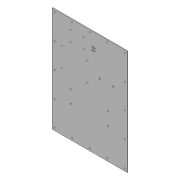
# Autodesk Inventor part: Board_Mounter
Saved by Autodesk Inventor 2020 (Build 240168000, 168)
## iProperties
Created: 2020-11-10
Part Number: Board_Mounter
Material: Generic
Document SubType Name: Modeling
Designer: magnarecta
Density: 1 g/cm^3
Appearance: Default
Author: magnarecta
Autodesk Inventor part; units mm, degrees
ref_plane "YZ Plane" through (0, 0, 0) normal (1, 0, 0) x (0, 1, 0)
ref_plane "XZ Plane" through (0, 0, 0) normal (0, 1, 0) x (-1, 0, 0)
ref_plane "XY Plane" through (0, 0, 0) normal (0, 0, 1) x (1, 0, 0)
sketch "Sketch2" plane through (0, 0, 0) normal (0, 0, 1) x (1, 0, 0)
  line L0 (150, -210) -> (-150, -210)
  line L1 (-150, -210) -> (-150, 210)
  line L2 (-150, 210) -> (150, 210)
  line L3 (150, 210) -> (150, -210)
  line L4 (150, -210) -> (-150, 210) construction
  line L5 (-150, -210) -> (150, 210) construction
  point P0 (0, 0)
  dimension "d4" = 420
  dimension "d5" = 300
  constraints: 12 end point, 2 midpoint, 2 parallel, 1 horizontal, 1 perpendicular
  measures "d4" distance of L2.end L0.start
  measures "d5" distance of L0.start L0.end
extrude "Extrusion2" add sketch "Sketch2" along normal blind 3
sketch "Sketch3" plane through (0, 0, 3) normal (0, 0, 1) x (1, 0, 0)
  line L0 (-150, 210) -> (-150, -210) projected
  line L1 (-150, -210) -> (150, -210) projected
  line L2 (150, -210) -> (150, 210) projected
  line L3 (150, 210) -> (-150, 210) projected
  line L4 (-140, 200) -> (-140, -200)
  line L5 (-140, -200) -> (140, -200)
  line L6 (140, -200) -> (140, 200)
  line L7 (140, 200) -> (-140, 200)
  point P0 (0, 0)
  point P1 (-70, 200)
  point P2 (-70, -200)
  point P3 (0, 200)
  point P4 (0, -200)
  point P5 (70, 200)
  point P6 (70, -200)
  dimension "d8" = 10
  dimension "d9" = 70
  dimension "d12" = 70
  constraints: 8 end point, 4 coincident, 2 point on line, 1 horizontal, 1 vertical alignment, 7 other
  measures "d8" distance between parallel lines of L3 L7
  measures "d9" distance from line of point (-70, 200) L4
  measures "d12" distance of point (-70, 200) point (0, 200)
hole "Hole1" at (-140, 200, 3) at (140, 200, 3) at (-140, -200, 3) at (140, -200, 3) at (-70, 200, 3) at (-70, -200, 3) at (0, 200, 3) at (70, 200, 3) at (70, -200, 3) at (0, -200, 3) direction (0, 0, -1) diameter 4.3 end through all
sketch "Sketch4" plane through (0, 0, 3) normal (0, 0, 1) x (1, 0, 0)
  line L0 (-75, -85) -> (75, -85)
  line L1 (75, -85) -> (75, -35)
  line L2 (75, -35) -> (-75, -35)
  line L3 (-75, -35) -> (-75, -85)
  line L4 (-75, -85) -> (75, -35) construction
  line L5 (75, -85) -> (-75, -35) construction
  line L6 (150, -210) -> (150, 210) projected
  line L7 (150, 210) -> (-150, 210) projected
  line L8 (-150, -210) -> (150, -210) projected
  point P0 (0, 0)
  point P1 (0, -60)
  dimension "d24" = 150
  dimension "d25" = 50
  dimension "d26" = 150
  dimension "d35" = 150
  constraints: 12 end point, 2 midpoint, 2 parallel, 1 horizontal, 1 perpendicular
  measures "d24" distance of L2.end L1.end
  measures "d25" distance of L1.end L0.end
  measures "d26" distance from line of L6 point (0, -60)
  measures "d35" distance from line of point (0, -60) L8
hole "Hole2" at (-75, -85, 3) at (-75, -35, 3) at (75, -85, 3) at (75, -35, 3) direction (0, 0, -1) diameter 4.3 end through all
sketch "Sketch5" plane through (0, 0, 3) normal (0, 0, 1) x (1, 0, 0)
  line L0 (-110.925, 21.95) -> (-9.075, 21.95)
  line L1 (-9.075, 21.95) -> (-9.075, 98.05)
  line L2 (-9.075, 98.05) -> (-110.925, 98.05)
  line L3 (-110.925, 98.05) -> (-110.925, 21.95)
  line L4 (-110.925, 21.95) -> (-9.075, 98.05) construction
  line L5 (-9.075, 21.95) -> (-110.925, 98.05) construction
  point P0 (0, 0)
  point P1 (-60, 60)
  dimension "d36" = 101.85
  dimension "d37" = 76.1
  dimension "d38" = 60
  dimension "d68" = 60
  constraints: 12 end point, 2 midpoint, 2 parallel, 1 horizontal, 1 perpendicular
  measures "d36" distance of L2.end L1.end
  measures "d37" distance of L1.end L0.end
  measures "d38" horizontal distance of point (-60, 60) point (0, 0)
  measures "d68" horizontal distance of point (-60, 60) point (0, 0)
hole "Hole3" at (-110.925, 98.05, 3) at (-110.925, 21.95, 3) at (-9.075, 21.95, 3) at (-9.075, 98.05, 3) direction (0, 0, -1) diameter 3.2 end through all
sketch "Sketch6" plane through (0, 0, 3) normal (0, 0, 1) x (1, 0, 0)
  line L0 (-24, 129) -> (-76, 129)
  line L1 (-76, 129) -> (-76, 171)
  line L2 (-76, 171) -> (-24, 171)
  line L3 (-24, 171) -> (-24, 129)
  line L4 (-24, 129) -> (-76, 171) construction
  line L5 (-76, 129) -> (-24, 171) construction
  point P0 (0, 0)
  point P1 (-50, 150)
  dimension "d48" = 52
  dimension "d49" = 42
  dimension "d50" = 150
  dimension "d51" = 50
  constraints: 12 end point, 2 midpoint, 2 parallel, 1 horizontal, 1 perpendicular
  measures "d48" distance of L1.end L2.end
  measures "d49" distance of L0.end L1.end
  measures "d50" vertical distance of point (-50, 150) point (0, 0)
  measures "d51" horizontal distance of point (-50, 150) point (0, 0)
hole "Hole4" at (-24, 129, 3) at (-24, 171, 3) at (-76, 129, 3) at (-76, 171, 3) direction (0, 0, -1) diameter 3.2 end through all
sketch "Sketch7" plane through (0, 0, 3) normal (0, 0, 1) x (1, 0, 0)
  circle A0 centre (-76, 129) radius 1.6 projected
  circle A1 centre (-24, 129) radius 1.6 projected
  circle A2 centre (-24, 171) radius 1.6 projected
  circle A3 centre (-76, 171) radius 1.6 projected
  circle A4 centre (-9.075, 21.95) radius 1.6 projected
  circle A5 centre (-110.925, 98.05) radius 1.6 projected
  circle A6 centre (-110.925, 21.95) radius 1.6 projected
  circle A7 centre (-9.075, 98.05) radius 1.6 projected
  circle A8 centre (75, -85) radius 2.15 projected
  circle A9 centre (-75, -85) radius 2.15 projected
  circle A10 centre (-75, -35) radius 2.15 projected
  circle A11 centre (75, -35) radius 2.15 projected
  circle A12 centre (70, -200) radius 2.15 projected
  circle A13 centre (0, 200) radius 2.15 projected
  circle A14 centre (-70, 200) radius 2.15 projected
  circle A15 centre (-140, -200) radius 2.15 projected
  circle A16 centre (-140, 200) radius 2.15 projected
  circle A17 centre (140, 200) radius 2.15 projected
  circle A18 centre (140, -200) radius 2.15 projected
  circle A19 centre (-70, -200) radius 2.15 projected
  circle A20 centre (70, 200) radius 2.15 projected
  circle A21 centre (0, -200) radius 2.15 projected
  line L0 (-150, 210) -> (-150, -210) projected
  line L1 (-150, -210) -> (150, -210) projected
  line L2 (150, -210) -> (150, 210) projected
  line L3 (150, 210) -> (-150, 210) projected
  circle A22 centre (-110.925, 21.95) radius 1.6 projected
  circle A23 centre (-110.925, 98.05) radius 1.6 projected
  line L4 (-110.925, 21.95) -> (-110.925, 98.05)
  point P0 (0, 0)
  point P1 (40, 60)
  point P2 (95, 60)
  point P3 (-110.925, 60)
  dimension "d59" = 55
  dimension "d69" = 40
  constraints: 2 end point, 2 horizontal alignment, 1 midpoint, 1 vertical
  measures "d59" distance of point (40, 60) point (95, 60)
  measures "d69" horizontal distance of point (40, 60) point (0, 0)
hole "Hole5" at (40, 60, 3) at (95, 60, 3) direction (0, 0, -1) diameter 5 end through all
sketch "Sketch8" plane through (0, 0, 3) normal (0, 0, 1) x (1, 0, 0)
  circle A0 centre (40, 60) radius 2.5 projected
  circle A1 centre (95, 60) radius 2.5 projected
  circle A2 centre (-76, 129) radius 1.6 projected
  circle A3 centre (-24, 129) radius 1.6 projected
  circle A4 centre (-24, 171) radius 1.6 projected
  circle A5 centre (-76, 171) radius 1.6 projected
  circle A6 centre (-9.075, 21.95) radius 1.6 projected
  circle A7 centre (-110.925, 98.05) radius 1.6 projected
  circle A8 centre (-110.925, 21.95) radius 1.6 projected
  circle A9 centre (-9.075, 98.05) radius 1.6 projected
  circle A10 centre (75, -85) radius 2.15 projected
  circle A11 centre (-75, -85) radius 2.15 projected
  circle A12 centre (-75, -35) radius 2.15 projected
  circle A13 centre (75, -35) radius 2.15 projected
  circle A14 centre (70, -200) radius 2.15 projected
  circle A15 centre (0, 200) radius 2.15 projected
  circle A16 centre (-70, 200) radius 2.15 projected
  circle A17 centre (-140, -200) radius 2.15 projected
  circle A18 centre (-140, 200) radius 2.15 projected
  circle A19 centre (140, 200) radius 2.15 projected
  circle A20 centre (140, -200) radius 2.15 projected
  circle A21 centre (-70, -200) radius 2.15 projected
  circle A22 centre (70, 200) radius 2.15 projected
  circle A23 centre (0, -200) radius 2.15 projected
  line L0 (-150, 210) -> (-150, -210) projected
  line L1 (-150, -210) -> (150, -210) projected
  line L2 (150, -210) -> (150, 210) projected
  line L3 (150, 210) -> (-150, 210) projected
  line L4 (-140, -200) -> (-140, 200)
  line L5 (-140, 200) -> (140, 200)
  line L6 (140, 200) -> (140, -200)
  line L7 (140, -200) -> (-140, -200)
  point P0 (0, 0)
  point P1 (-140, 0)
  point P2 (-140, -100)
  point P3 (-140, 100)
  point P4 (140, 100)
  point P5 (140, 0)
  point P6 (140, -100)
  dimension "d26" = 150
  dimension "d70" = 10
  dimension "d71" = 100
  dimension "d72" = 100
  constraints: 8 end point, 4 point on line, 2 horizontal alignment, 2 midpoint, 3 other
  measures "d70" distance between parallel lines of L0 L4
  measures "d71" distance from line of point (-140, -100) L7
  measures "d72" distance of point (-140, 100) point (-140, 0)
hole "Hole6" at (-140, 0, 3) at (-140, -100, 3) at (-140, 100, 3) at (140, 100, 3) at (140, 0, 3) at (140, -100, 3) direction (0, 0, -1) diameter 4.2 end through all
sketch "Sketch9" plane through (0, 0, 3) normal (0, 0, 1) x (1, 0, 0)
  circle A0 centre (140, 0) radius 2.1 projected
  circle A1 centre (-140, 100) radius 2.1 projected
  circle A2 centre (-140, 0) radius 2.1 projected
  circle A3 centre (-140, -100) radius 2.1 projected
  circle A4 centre (140, 100) radius 2.1 projected
  circle A5 centre (140, -100) radius 2.1 projected
  circle A6 centre (40, 60) radius 2.5 projected
  circle A7 centre (95, 60) radius 2.5 projected
  circle A8 centre (-76, 129) radius 1.6 projected
  circle A9 centre (-24, 129) radius 1.6 projected
  circle A10 centre (-24, 171) radius 1.6 projected
  circle A11 centre (-76, 171) radius 1.6 projected
  circle A12 centre (-9.075, 21.95) radius 1.6 projected
  circle A13 centre (-110.925, 98.05) radius 1.6 projected
  circle A14 centre (-110.925, 21.95) radius 1.6 projected
  circle A15 centre (-9.075, 98.05) radius 1.6 projected
  circle A16 centre (75, -85) radius 2.15 projected
  circle A17 centre (-75, -85) radius 2.15 projected
  circle A18 centre (-75, -35) radius 2.15 projected
  circle A19 centre (75, -35) radius 2.15 projected
  circle A20 centre (70, -200) radius 2.15 projected
  circle A21 centre (0, 200) radius 2.15 projected
  circle A22 centre (-70, 200) radius 2.15 projected
  circle A23 centre (-140, -200) radius 2.15 projected
  circle A24 centre (-140, 200) radius 2.15 projected
  circle A25 centre (140, 200) radius 2.15 projected
  circle A26 centre (140, -200) radius 2.15 projected
  circle A27 centre (-70, -200) radius 2.15 projected
  circle A28 centre (70, 200) radius 2.15 projected
  circle A29 centre (0, -200) radius 2.15 projected
  line L0 (-150, 210) -> (-150, -210) projected
  line L1 (-150, -210) -> (150, -210) projected
  line L2 (150, -210) -> (150, 210) projected
  line L3 (150, 210) -> (-150, 210) projected
  line L4 (11.125, 145) -> (20.875, 145) construction
  line L5 (11.125, 143.5) -> (20.875, 143.5)
  line L6 (20.875, 146.5) -> (11.125, 146.5)
  arc A30 (11.125, 146.5) -> (11.125, 143.5) centre (11.125, 145) ccw
  arc A31 (20.875, 143.5) -> (20.875, 146.5) centre (20.875, 145) ccw
  line L7 (20.875, 155) -> (11.125, 155) construction
  line L8 (20.875, 156.5) -> (11.125, 156.5)
  line L9 (11.125, 153.5) -> (20.875, 153.5)
  arc A32 (20.875, 153.5) -> (20.875, 156.5) centre (20.875, 155) ccw
  arc A33 (11.125, 156.5) -> (11.125, 153.5) centre (11.125, 155) ccw
  circle A34 centre (-24, 129) radius 1.6 projected
  circle A35 centre (-24, 171) radius 1.6 projected
  line L10 (-24, 129) -> (-24, 171)
  point P0 (0, 0)
  point P1 (16, 145)
  point P2 (16, 155)
  point P3 (-24, 150)
  dimension "d80" = 1.5
  dimension "d81" = 1.5
  dimension "d82" = 10
  dimension "d83" = 5
  dimension "d84" = 40
  constraints: 18 end point, 8 point on circle, 8 tangent, 4 centre point, 3 midpoint, 3 parallel, 2 vertical alignment, 1 horizontal, 1 vertical
  measures "d80" radius of A32
  measures "d81" radius of A31
  measures "d82" distance between parallel lines of L7 L4
  measures "d83" distance from line of L7 point (-24, 150)
  measures "d84" distance from line of point (16, 155) L10
extrude "Extrusion3" cut sketch "Sketch9" against normal blind 3 contours A30 L6 A31 L5 | A32 L9 A33 L8
body "Solid2"
